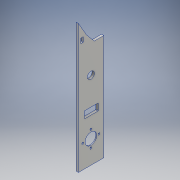
# Autodesk Inventor part: 옆판_왼쪽
Saved by Autodesk Inventor 2017 (Build 210142000, 142)
## iProperties
Part Number: 옆판_왼쪽
Material: 알루미늄 6061
Document SubType Name: Modeling
Designer: minom
Density: 2.7 g/cm^3
Appearance: 알루미늄 - 평지
Mass: 118.35 g
Surface Area: 319.268 cm^2
Volume: 43.8332 cm^3
Author: minom
Autodesk Inventor part; units mm, degrees
ref_plane "YZ Plane" through (0, 0, 0) normal (1, 0, 0) x (0, 1, 0)
ref_plane "XZ Plane" through (0, 0, 0) normal (0, 1, 0) x (-1, 0, 0)
ref_plane "XY Plane" through (0, 0, 0) normal (0, 0, 1) x (1, 0, 0)
sketch "스케치1" plane through (0, 0, 0) normal (1, 0, 0) x (0, 1, 0)
  line L0 (-1.6916, -0.1268) -> (-1.6916, 279.8732)
  line L1 (-1.6916, 279.8732) -> (53.3084, 279.8732)
  line L2 (53.3084, 279.8732) -> (53.3084, -0.1268)
  line L3 (53.3084, -0.1268) -> (-1.6916, -0.1268)
  line L4 (-1.6916, 279.8732) -> (-1.6916, 249.8732)
  line L5 (-1.6916, 249.8732) -> (-1.6916, 229.8732)
  line L6 (-1.6916, 229.8732) -> (-1.6916, 220)
  line L7 (-1.6916, 229.8732) -> (53.3084, 229.8732)
  line L8 (-1.6916, 249.8732) -> (53.3084, 249.8732)
  line L9 (-1.6916, 279.8732) -> (15.6289, 249.8732)
  line L10 (-1.6916, 279.8732) -> (32.9494, 279.8732) construction
  line L11 (15.6289, 249.8732) -> (32.4109, 229.8732)
  line L12 (15.6289, 249.8732) -> (41.737, 249.8732) construction
  line L13 (32.4109, 229.8732) -> (47.1107, 229.8732) construction
  point P0 (0, 0)
  point P1 (53.3084, 219.8732)
  dimension "d0" = 280
  dimension "d1" = 55
  dimension "d2" = 30
  dimension "d3" = 20
  dimension "d4" = 60
  dimension "d5" = 50
  constraints: 28 end point, 8 point on line, 5 perpendicular, 3 horizontal, 2 equal length, 1 vertical
  measures "d0" distance of L3.end L4.start
  measures "d1" distance of L4.start L1.end
  measures "d2" distance of L4.start L8.start
  measures "d3" distance of L8.start L6.start
  measures "d4" angle of L9 L10
  measures "d5" angle of L11 L12
extrude "돌출1" add sketch "스케치1" along normal blind 5 contours L0 L7 L2 L3 | L0 L8 L11 L7 | L0 L9 L8
sketch "스케치3" plane through (0, 0, 0) normal (-1, 0, 0) x (0, 0, 1)
  circle A0 centre (49.8732, 25.3084) radius 21.25
  line L0 (279.8732, -1.6916) -> (-0.1268, -1.6916) projected
  line L1 (-0.1268, -1.6916) -> (49.8732, -1.6916)
  line L2 (49.8732, -1.6916) -> (49.8732, 25.3084)
  point P0 (0, 0)
  dimension "d13" = 42.5
  dimension "d139" = 50
  dimension "d140" = 27
  constraints: 4 end point, 1 centre point, 1 coincident, 1 perpendicular, 1 point on line
  measures "d13" diameter of A0
  measures "d139" distance of L0.end L1.end
  measures "d140" distance of L1.end L2.end
extrude "돌출2" cut sketch "스케치3" against normal blind 3
sketch "스케치4" plane through (3, 25.3084, 49.8732) normal (-1, 0, 0) x (0, 0, 1)
  circle A0 centre (0, 0) radius 12.6
  point P0 (-49.8732, -25.3084)
  dimension "d16" = 25.2
  constraints: 1 centre point
  measures "d16" diameter of A0
extrude "돌출3" cut sketch "스케치4" against normal blind 3
sketch "스케치5" plane through (3, 25.3084, 49.8732) normal (-1, 0, 0) x (0, 0, 1)
  circle A0 centre (0, 17.6) radius 2.1
  circle A1 centre (17.6, 0) radius 2.1
  circle A2 centre (0, -17.6) radius 2.1
  circle A3 centre (-17.6, 0) radius 2.1
  point P0 (-49.8732, -25.3084)
  dimension "d20" = 4.2
  dimension "d24" = 4.2
  dimension "d25" = 4.2
  dimension "d26" = 4.2
  constraints: 4 centre point
  measures "d20" diameter of A0
  measures "d24" diameter of A1
  measures "d25" diameter of A2
  measures "d26" diameter of A3
extrude "돌출4" cut sketch "스케치5" against normal blind 3
sketch "스케치6" plane through (5, 0, 0) normal (1, 0, 0) x (0, 0, -1)
  circle A0 centre (-49.8732, 25.3084) radius 12.6 projected
  line L0 (-49.8732, 25.3084) -> (-169.2232, 25.3084)
  circle A1 centre (-169.2232, 25.3084) radius 7.55
  point P0 (0, 0)
  dimension "d29" = 119.35
  dimension "d30" = 15.1
  constraints: 2 end point, 1 centre point, 1 coincident, 1 horizontal
  measures "d29" distance of L0.start L0.end
  measures "d30" diameter of A1
extrude "돌출5" cut sketch "스케치6" against normal blind 5 contours A1
sketch "스케치7" plane through (0, 0, 0) normal (-1, 0, 0) x (0, 0, 1)
  circle A0 centre (169.2232, 25.3084) radius 7.55 projected
  circle A1 centre (49.8732, 25.3084) radius 21.25 projected
  line L0 (279.8732, -1.6916) -> (-0.1268, -1.6916) projected
  line L1 (249.8732, 15.6289) -> (279.8732, -1.6916) projected
  line L2 (229.8732, 32.4109) -> (249.8732, 15.6289) projected
  line L3 (229.8732, 53.3084) -> (229.8732, 32.4109) projected
  line L4 (-0.1268, 53.3084) -> (229.8732, 53.3084) projected
  line L5 (-0.1268, -1.6916) -> (-0.1268, 53.3084) projected
  line L6 (169.2232, 25.3084) -> (109.2232, 25.3084)
  line L7 (96.8732, 53.3084) -> (96.8732, 41.3084)
  line L8 (96.8732, 41.3084) -> (108.2232, 41.3084)
  line L9 (109.2232, 40.3084) -> (109.2232, 25.3084)
  line L10 (109.2232, 25.3084) -> (109.2232, 12.3084)
  line L11 (108.2232, 11.3084) -> (95.2232, 11.3084)
  line L12 (94.2232, 12.3084) -> (94.2232, 40.3084)
  line L13 (49.8732, 25.3084) -> (94.2232, 26.3084)
  line L14 (96.8732, 41.3084) -> (95.2232, 41.3084)
  arc A2 (95.2232, 41.3084) -> (94.2232, 40.3084) centre (95.2232, 40.3084) ccw
  arc A3 (109.2232, 40.3084) -> (108.2232, 41.3084) centre (108.2232, 40.3084) ccw
  arc A4 (108.2232, 11.3084) -> (109.2232, 12.3084) centre (108.2232, 12.3084) ccw
  arc A5 (94.2232, 12.3084) -> (95.2232, 11.3084) centre (95.2232, 12.3084) ccw
  point P0 (0, 0)
  point P1 (109.2232, 11.3084)
  point P2 (94.2232, 11.3084)
  dimension "d33" = 60
  dimension "d34" = 12
  dimension "d35" = 14
  dimension "d36" = 15
  dimension "d37" = 1
  constraints: 18 end point, 8 point on circle, 8 tangent, 5 point on line, 4 centre point, 4 perpendicular, 3 equal radius, 2 horizontal, 2 vertical, 1 midpoint
  measures "d33" distance of L6.start L6.end
  measures "d34" distance of L7.start L7.end
  measures "d35" distance of L6.end point (109.223, 11.308)
  measures "d36" distance of point (109.223, 11.308) point (94.223, 11.308)
  measures "d37" radius of A2
extrude "돌출6" cut sketch "스케치7" against normal blind 10 contours L10 A4 L11 A5 L12 A2 L14 L8 A3 L9
sketch "스케치8" plane through (0, 0, 0) normal (-1, 0, 0) x (0, 0, 1)
  arc A0 (95.2232, 41.3084) -> (94.2232, 40.3084) centre (95.2232, 40.3084) ccw projected
  line L0 (95.2232, 41.3084) -> (108.2232, 41.3084) projected
  arc A1 (109.2232, 40.3084) -> (108.2232, 41.3084) centre (108.2232, 40.3084) ccw projected
  line L1 (109.2232, 40.3084) -> (109.2232, 12.3084) projected
  arc A2 (108.2232, 11.3084) -> (109.2232, 12.3084) centre (108.2232, 12.3084) ccw projected
  line L2 (108.2232, 11.3084) -> (95.2232, 11.3084) projected
  arc A3 (94.2232, 12.3084) -> (95.2232, 11.3084) centre (95.2232, 12.3084) ccw projected
  line L3 (94.2232, 12.3084) -> (94.2232, 40.3084) projected
  circle A4 centre (169.2232, 25.3084) radius 7.55 projected
  circle A5 centre (49.8732, 25.3084) radius 21.25 projected
  line L4 (279.8732, -1.6916) -> (-0.1268, -1.6916) projected
  line L5 (249.8732, 15.6289) -> (279.8732, -1.6916) projected
  line L6 (229.8732, 32.4109) -> (249.8732, 15.6289) projected
  line L7 (229.8732, 53.3084) -> (229.8732, 32.4109) projected
  line L8 (-0.1268, 53.3084) -> (229.8732, 53.3084) projected
  line L9 (-0.1268, -1.6916) -> (-0.1268, 53.3084) projected
  line L10 (109.2232, 40.3084) -> (109.2232, 12.3084) projected
  line L11 (109.2232, 26.3084) -> (113.2232, 26.3084)
  line L12 (94.2232, 26.3084) -> (90.2232, 26.3084)
  line L13 (-0.1268, 53.3084) -> (229.8732, 53.3084) projected
  line L14 (249.8732, 15.6289) -> (279.8732, -1.6916) projected
  line L15 (-0.1268, 0) -> (-0.1268, 53.3084) projected
  line L16 (21.3373, 48.3084) -> (32.5076, 48.3084) construction
  line L17 (21.3373, 3.3084) -> (30.282, 3.3084) construction
  line L18 (21.0776, 44.1489) -> (27.4785, 40.4533)
  line L19 (21.0776, 44.1489) -> (20.3373, 44.5763)
  line L20 (25.4995, 36.9771) -> (12.8732, 44.2669)
  line L21 (19.0776, 40.6848) -> (25.4995, 36.9771)
  line L22 (81.4518, 40.9348) -> (74.3109, 36.812)
  line L23 (81.4518, 40.9348) -> (87.2232, 44.2669)
  line L24 (79.0188, 44.1489) -> (72.3768, 40.3142)
  line L25 (79.0188, 44.1489) -> (79.7591, 44.5763)
  line L26 (79.7591, 7.0404) -> (72.9016, 10.9996)
  line L27 (83.2036, 9.6705) -> (87.2232, 7.3498)
  line L28 (83.2036, 9.6705) -> (74.6129, 14.6304)
  line L29 (20.3373, 7.0404) -> (26.9488, 10.8576)
  line L30 (17.7104, 10.1426) -> (25.1925, 14.4624)
  line L31 (17.7104, 10.1426) -> (12.8732, 7.3498)
  arc A6 (67.0232, 6.7763) -> (70.2849, 10.4448) centre (49.8732, 25.3084) ccw
  line L32 (78.7591, 3.3084) -> (68.3816, 3.3084)
  line L33 (90.2232, 26.3084) -> (90.2232, 9.0819)
  arc A7 (73.7237, 17.019) -> (73.4439, 34.3628) centre (49.8732, 25.3084) ccw
  arc A8 (69.7985, 40.8178) -> (65.9642, 44.7671) centre (49.8732, 25.3084) ccw
  arc A9 (33.7821, 44.7671) -> (30.0488, 40.9467) centre (49.8732, 25.3084) ccw
  arc A10 (26.3617, 34.5158) -> (26.0773, 16.8633) centre (49.8732, 25.3084) ccw
  arc A11 (29.5579, 10.3133) -> (32.7231, 6.7763) centre (49.8732, 25.3084) ccw
  line L34 (9.8732, 25.8084) -> (9.8732, 9.0819)
  line L35 (31.3647, 3.3084) -> (21.3373, 3.3084)
  line L36 (9.8732, 25.8084) -> (9.8732, 42.5349)
  line L37 (90.2232, 26.3084) -> (90.2232, 42.5349)
  line L38 (78.7591, 48.3084) -> (67.2387, 48.3084)
  arc A12 (12.8732, 44.2669) -> (9.8732, 42.5349) centre (11.8732, 42.5349) ccw
  arc A13 (26.3617, 34.5158) -> (25.4995, 36.9771) centre (24.4995, 35.2451) ccw
  arc A14 (25.1925, 14.4624) -> (26.0773, 16.8633) centre (24.1925, 16.1944) ccw
  arc A15 (9.8732, 9.0819) -> (12.8732, 7.3498) centre (11.8732, 9.0819) ccw
  arc A16 (20.3373, 7.0404) -> (21.3373, 3.3084) centre (21.3373, 5.3084) ccw
  arc A17 (31.3647, 3.3084) -> (32.7231, 6.7763) centre (31.3647, 5.3084) ccw
  arc A18 (29.5579, 10.3133) -> (26.9488, 10.8576) centre (27.9488, 9.1255) ccw
  arc A19 (21.3373, 48.3084) -> (20.3373, 44.5763) centre (21.3373, 46.3084) ccw
  arc A20 (33.7821, 44.7671) -> (32.5076, 48.3084) centre (32.5076, 46.3084) ccw
  arc A21 (27.4785, 40.4533) -> (30.0488, 40.9467) centre (28.4785, 42.1854) ccw
  arc A22 (67.2387, 48.3084) -> (65.9642, 44.7671) centre (67.2387, 46.3084) ccw
  arc A23 (79.7591, 44.5763) -> (78.7591, 48.3084) centre (78.7591, 46.3084) ccw
  arc A24 (69.7985, 40.8178) -> (72.3768, 40.3142) centre (71.3768, 42.0462) ccw
  arc A25 (74.3109, 36.812) -> (73.4439, 34.3628) centre (75.3109, 35.08) ccw
  arc A26 (73.7237, 17.019) -> (74.6129, 14.6304) centre (75.6129, 16.3624) ccw
  arc A27 (87.2232, 7.3498) -> (90.2232, 9.0819) centre (88.2232, 9.0819) ccw
  arc A28 (90.2232, 42.5349) -> (87.2232, 44.2669) centre (88.2232, 42.5349) ccw
  arc A29 (78.7591, 3.3084) -> (79.7591, 7.0404) centre (78.7591, 5.3084) ccw
  arc A30 (67.0232, 6.7763) -> (68.3816, 3.3084) centre (68.3816, 5.3084) ccw
  arc A31 (72.9016, 10.9996) -> (70.2849, 10.4448) centre (71.9016, 9.2675) ccw
  line L39 (21.3373, 48.3084) -> (32.5076, 48.3084)
  line L40 (-0.1268, 53.3084) -> (229.8732, 53.3084) projected
  line L41 (249.8732, 15.6289) -> (279.8732, -1.6916) projected
  line L42 (113.2232, 26.3084) -> (113.2232, 42.5426)
  line L43 (113.2232, 26.3084) -> (113.2232, 9.0896)
  line L44 (168.2114, 48.3161) -> (124.6873, 48.3161)
  line L45 (168.2114, 48.3161) -> (209.9814, 48.0944)
  line L46 (279.8732, -1.6916) -> (-0.1268, -1.6916) projected
  circle A32 centre (169.2232, 25.3084) radius 7.55 projected
  line L47 (221.8732, 42.3105) -> (221.8732, 9.0818)
  line L48 (134.6273, 33.649) -> (116.2232, 44.2747)
  line L49 (136.6273, 37.1131) -> (151.1943, 28.7029)
  line L50 (136.6273, 37.1131) -> (123.6873, 44.5841)
  line L51 (127.8049, 14.0443) -> (116.2232, 7.3576)
  line L52 (129.8049, 10.5802) -> (123.6873, 7.0482)
  line L53 (129.8049, 10.5802) -> (151.1938, 22.9368)
  line L54 (201.9585, 34.5406) -> (218.8936, 44.0542)
  line L55 (199.9994, 38.028) -> (210.9708, 44.3624)
  line L56 (199.9994, 38.028) -> (183.0579, 28.5832)
  line L57 (199.9334, 13.4173) -> (211.0142, 7.0419)
  line L58 (199.9334, 13.4173) -> (183.06, 22.8392)
  line L59 (201.9519, 16.8707) -> (218.8924, 7.3388)
  line L60 (127.8049, 14.0443) -> (145.1943, 24.0841)
  line L61 (153.1957, 28.7036) -> (160.5888, 32.9798)
  line L62 (134.6273, 33.649) -> (145.1943, 27.5482)
  line L63 (153.1943, 22.9371) -> (158.853, 19.67)
  arc A33 (159.5313, 19.0258) -> (180.2032, 21.7248) centre (169.2232, 25.3084) ccw
  arc A34 (179.8781, 29.7666) -> (160.5888, 32.9798) centre (169.2232, 25.3084) ccw
  line L64 (201.9585, 34.5406) -> (189.2281, 27.1907)
  line L65 (181.0849, 22.8251) -> (181.1045, 22.8364)
  line L66 (201.9519, 16.8707) -> (189.2795, 23.6979)
  line L67 (181.0841, 28.5981) -> (180.7231, 28.8065)
  arc A35 (124.6873, 48.3161) -> (123.6873, 44.5841) centre (124.6873, 46.3161) ccw
  arc A36 (116.2232, 44.2747) -> (113.2232, 42.5426) centre (115.2232, 42.5426) ccw
  arc A37 (113.2232, 9.0896) -> (116.2232, 7.3576) centre (115.2232, 9.0896) ccw
  arc A38 (145.1943, 24.0841) -> (145.1943, 27.5482) centre (144.1943, 25.8161) ccw
  arc A39 (151.1943, 28.7029) -> (153.1957, 28.7036) centre (152.1943, 30.4349) ccw
  arc A40 (153.1943, 22.9371) -> (151.1938, 22.9368) centre (152.1943, 21.205) ccw
  arc A41 (123.6873, 7.0482) -> (124.6869, 3.3161) centre (124.6873, 5.3161) ccw
  arc A42 (159.5313, 19.0258) -> (158.853, 19.67) centre (157.853, 17.938) ccw
  arc A43 (181.1045, 22.8364) -> (180.2032, 21.7248) centre (182.1045, 21.1043) ccw
  arc A44 (179.8781, 29.7666) -> (180.7231, 28.8065) centre (181.7231, 30.5385) ccw
  arc A45 (181.0841, 28.5981) -> (183.0579, 28.5832) centre (182.0841, 30.3301) ccw
  arc A46 (210.9708, 44.3624) -> (209.9814, 48.0944) centre (209.9708, 46.0944) ccw
  arc A47 (221.8732, 42.3105) -> (218.8936, 44.0542) centre (219.8732, 42.3105) ccw
  arc A48 (189.2281, 27.1907) -> (189.2795, 23.6979) centre (190.2281, 25.4587) ccw
  arc A49 (183.06, 22.8392) -> (181.0849, 22.8251) centre (182.0849, 21.093) ccw
  arc A50 (218.8924, 7.3388) -> (221.8732, 9.0818) centre (219.8732, 9.0818) ccw
  arc A51 (210.0168, 3.3084) -> (211.0142, 7.0419) centre (210.0168, 5.3084) ccw
  line L68 (169.2231, 3.3084) -> (210.0168, 3.3084)
  line L69 (124.6869, 3.3161) -> (169.2231, 3.3084)
  point P0 (0, 0)
  point P1 (29.0285, 39.5584)
  point P2 (72.781, 35.9288)
  point P3 (90.2232, 45.999)
  point P4 (86.2232, 48.3084)
  point P5 (71.2883, 11.931)
  point P6 (86.2232, 3.3084)
  point P7 (26.6818, 15.3222)
  point P8 (9.8732, 5.6178)
  point P9 (60.2925, 48.3084)
  point P10 (62.2652, 3.3084)
  point P11 (37.4811, 3.3084)
  point P12 (73.1337, 15.4844)
  point P13 (70.8163, 39.4132)
  point P14 (28.5513, 11.7828)
  point P15 (271.2129, 3.3084)
  point P16 (159.2873, 19.4193)
  point P17 (180.1124, 29.1591)
  point P18 (180.4102, 22.4355)
  point P19 (181.0947, 22.8307)
  dimension "d40" = 4
  dimension "d41" = 4
  dimension "d53" = 4
  dimension "d60" = 2
  dimension "d61" = 2
  dimension "d62" = 2
  dimension "d78" = 4
  dimension "d79" = 4
  dimension "d85" = 4
  dimension "d121" = 4
  dimension "d127" = 4
  dimension "d129" = 4
  dimension "d131" = 4
  dimension "d134" = 2
  dimension "d135" = 8
  dimension "d136" = 5
  constraints: 106 end point, 105 point on circle, 71 tangent, 45 centre point, 33 equal radius, 30 point on line, 7 parallel, 7 perpendicular, 4 horizontal, 2 coincident, 2 collinear, 2 midpoint, 2 vertical, 1 other
  measures "d40" distance of L11.start L11.end
  measures "d41" distance of L12.start L12.end
  measures "d53" distance of L21.start L18.start
  measures "d60" radius of A12
  measures "d61" radius of A16
  measures "d62" radius of A19
  measures "d78" distance between parallel lines of L28 L26
  measures "d79" distance between parallel lines of L29 L30
  measures "d85" distance between parallel lines of L22 L24
  measures "d121" distance of L49.start L48.start
  measures "d127" distance of L52.start L51.start
  measures "d129" distance of L55.start L54.start
  measures "d131" distance of L59.start L57.start
  measures "d134" radius of A35
  measures "d135" distance between parallel lines of L7 L47
  measures "d136" distance between parallel lines of L4 L68
extrude "돌출9" cut sketch "스케치8" against normal blind 3 contours L42 A36 L48 L62 A38 L60 L51 A37 L43 | L33 A27 L27 L28 A26 A7 A25 L22 L23 A28 L37 | L19 A19 L39 A20 A9 A21 L18 | A13 A10 A14 L30 L31 A15 L34 L36 A12 L20 | L24 A24 A8 A22 L38 A23 L25 | A29 L32 A30 A6 A31 L26 | L29 A18 A11 A17 L35 A16 | L45 A46 L55 L56 A45 L67 A44 A34 L61 A39 L49 L50 A35 L44 | L47 A50 L59 L66 A48 L64 L54 A47 | L53 A40 L63 A42 A33 A43 L65 A49 L58 L57 A51 L68 L69 A41 L52
sketch "스케치9" plane through (0, 0, 0) normal (-1, 0, 0) x (0, 0, 1)
  line L0 (229.8732, 53.3084) -> (229.8732, 32.4109) projected
  line L1 (229.8732, 32.4109) -> (229.8732, -1.6916)
  line L2 (279.8732, -1.6916) -> (-0.1268, -1.6916) projected
  line L3 (229.8732, -1.6916) -> (249.8732, -1.6916)
  line L4 (249.8732, -1.6916) -> (249.8732, 3.3084)
  line L5 (248.8732, 3.3084) -> (240.3732, 3.3084)
  line L6 (239.3732, 4.3084) -> (239.3732, 7.8084)
  line L7 (240.3732, 8.8084) -> (248.8732, 8.8084)
  line L8 (249.8732, 7.8084) -> (249.8732, 4.3084)
  arc A0 (240.3732, 8.8084) -> (239.3732, 7.8084) centre (240.3732, 7.8084) ccw
  arc A1 (239.3732, 4.3084) -> (240.3732, 3.3084) centre (240.3732, 4.3084) ccw
  arc A2 (248.8732, 3.3084) -> (249.8732, 4.3084) centre (248.8732, 4.3084) ccw
  arc A3 (249.8732, 7.8084) -> (248.8732, 8.8084) centre (248.8732, 7.8084) ccw
  point P0 (0, 0)
  point P1 (239.3732, 8.8084)
  point P2 (239.3732, 3.3084)
  point P3 (249.8732, 8.8084)
  dimension "d141" = 20
  dimension "d142" = 5
  dimension "d143" = 10.5
  dimension "d144" = 5.5
  dimension "d145" = 1
  constraints: 14 end point, 10 point on line, 8 point on circle, 8 tangent, 4 centre point, 3 equal radius, 2 parallel, 2 perpendicular, 1 horizontal, 1 vertical
  measures "d141" distance of L1.end L3.end
  measures "d142" distance of L3.end L4.end
  measures "d143" distance of point (239.373, 8.808) point (249.873, 8.808)
  measures "d144" distance of point (239.373, 3.308) point (239.373, 8.808)
  measures "d145" radius of A0
extrude "돌출10" cut sketch "스케치9" against normal blind 10
